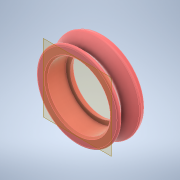
# Autodesk Inventor part: vroller
Saved by Autodesk Inventor 2022 (Build 260153000, 153)
## iProperties
Created: 2022-03-17
Part Number: vroller
Material: ABS Plastic
Document SubType Name: Modeling
Designer: zac-h
Density: 1.06 g/cm^3
Appearance: Smooth - Red
Author: zac-h
## iProperties of the stored document vroller_3DPrint.ipt
Created: 2022-03-17
Part Number: vroller_3DPrint
Material: Generic
Document SubType Name: Modeling
Designer: zac-h
Density: 1 g/cm^3
Appearance: Default
Author: zac-h
Autodesk Inventor part; units mm, degrees
ref_plane "YZ Plane" through (0, 0, 0) normal (1, 0, 0) x (0, 1, 0)
ref_plane "XZ Plane" through (0, 0, 0) normal (0, 1, 0) x (-1, 0, 0)
ref_plane "XY Plane" through (0, 0, 0) normal (0, 0, 1) x (1, 0, 0)
ref_plane "Work Plane1" through (0, 0, 0) normal (0, 0, 1) x (1, 0, 0)
sketch "Sketch1" plane through (0, 0, 0) normal (0, 1, 0) x (-1, 0, 0)
  line L0 (-11.125, -7) -> (11.125, -7)
  line L1 (11.125, -7) -> (11.125, 0)
  line L2 (11.125, 0) -> (-11.125, 0)
  line L3 (-11.125, 0) -> (-11.125, -7)
  line L4 (-11.125, -7) -> (11.125, 0) construction
  line L5 (11.125, -7) -> (-11.125, 0) construction
  line L6 (0, -3.5) -> (0, 0) construction
  line L7 (-11.125, 0) -> (-15.55, 0)
  line L8 (-15.55, 0) -> (-12.125, -3.425)
  line L9 (-12.125, -3.575) -> (-15.55, -7)
  line L10 (-15.55, -7) -> (-11.125, -7) construction
  line L11 (-12.125, -3.425) -> (-12.125, -3.575)
  line L12 (-15.55, -7) -> (-14.8221, -9)
  line L13 (-14.8221, -9) -> (-10.2279, -9)
  line L14 (-10.2279, -9) -> (-9.5, -7)
  dimension "d0" = 22.25
  dimension "d1" = 7
  dimension "d3" = 45
  dimension "d4" = 45
  dimension "d6" = 70
  dimension "d7" = 2
  dimension "d8" = 19
  dimension "d9" = 70
  dimension "d16" = 1
  dimension "d17" = 31.1
  constraints: 31 end point, 3 horizontal, 3 midpoint, 2 parallel, 2 perpendicular, 2 point on line, 1 coincident, 1 vertical
  measures "d0" distance of L2.end L1.end
  measures "d1" distance of L1.end L0.end
  measures "d3" angle of L7 L8
  measures "d4" angle of L10 L9
  measures "d6" angle of L10 L12
  measures "d7" distance between parallel lines of L10 L13
  measures "d8" diameter of L14.end L6
  measures "d9" angle of L0 L14
  measures "d16" distance between parallel lines of L3 L11
  measures "d17" diameter of L7.end L6
revolve "Revolution1" add sketch "Sketch1" angle 360 about axis through (0, 0, -3.5) along (0, 0, 1) contours L0 L14 L13 L12 L9 L11 L8 L7 L3
fillet "Fillet1" radius 0.6 4 edges at (-15.55, 0, 0) (-15.55, 0, -7) (-14.8221, 0, -9) (-10.2279, 0, -9)
chamfer "Chamfer1" distance 0.6 angle 45 1 edges at (-11.125, 0, 0)
body "Solid1"
